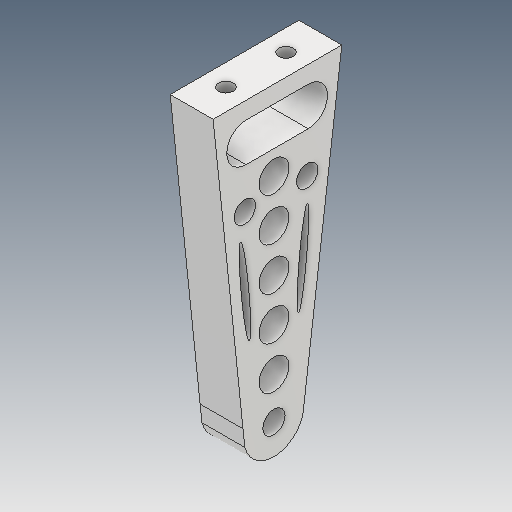
# Autodesk Inventor part: Radaufhängung
Saved by Autodesk Inventor 2018 (Build 220112000, 112)
## iProperties
Created: 2018-01-29
Part Number: Radaufhängung
Material: PC/ABS-Kunststoff
Document SubType Name: Modeling
Designer: Chris
Density: 0.357273 g/cm^3
Appearance: Schnee
Mass: 3.80196 g
Surface Area: 70.8958 cm^2
Volume: 10.6416 cm^3
Author: Chris
Autodesk Inventor part; units mm, degrees
note: some values were not read from the file. Chosen so that the rebuilt part matches the saved one: sketch regions of "Extrusion1".
ref_plane "YZ Plane" through (0, 0, 0) normal (1, 0, 0) x (0, 1, 0)
ref_plane "XZ Plane" through (0, 0, 0) normal (0, 1, 0) x (-1, 0, 0)
ref_plane "XY Plane" through (0, 0, 0) normal (0, 0, 1) x (1, 0, 0)
sketch "Skizze1" plane through (0, 0, 0) normal (1, 0, 0) x (0, 1, 0)
  line L0 (0, 0) -> (30, 0)
  line L1 (14.175552, 0) -> (14.175552, -68.187879) construction
  circle A0 centre (14.175552, -68.187879) radius 2.6
  circle A1 centre (14.175552, -68.187879) radius 7
  line L2 (0, 0) -> (7.179577, -67.95054)
  circle A2 centre (14.175552, -18.569993) radius 3.5
  arc A3 (7.675552, -4) -> (7.675552, -13) centre (7.675552, -8.5) ccw
  circle A4 centre (14.175552, -28.569993) radius 3.5
  circle A5 centre (14.175552, -38.569993) radius 3.5
  circle A6 centre (14.175552, -48.569993) radius 3.5
  circle A7 centre (14.175552, -58.569993) radius 3.5
  circle A8 centre (21.920836, -22.373144) radius 2.5
  circle A9 centre (7.389695, -22.35367) radius 2.5
  line L3 (7.675552, -4) -> (14.175552, -4)
  line L4 (7.675552, -13) -> (14.175552, -13)
  ellipse E0 centre (20.928749, -38.468301) end of major axis (19.90015, -48.968019) minor radius 0.865905
  ellipse E1 centre (7.422355, -38.468301) end of major axis (8.450954, -48.968019) minor radius 0.865905
  line L5 (21.175549, -68.194766) -> (30, 0)
  arc A10 (22.175552, -13) -> (22.175552, -4) centre (22.175552, -8.5) ccw
  line L6 (14.175552, -4) -> (22.175552, -4)
  line L7 (14.175552, -13) -> (22.175552, -13)
  point P0 (11.380257, -37.526628)
  point P1 (20.96203, -66.472155)
  dimension "d0" = 30
  dimension "d32" = 70
  dimension "d34" = 5.2
  dimension "d35" = 14
  dimension "d36" = 7
  dimension "d42" = 9
  dimension "d43" = 8.5
  dimension "d44" = 6.5
  dimension "d47" = 10
  dimension "d54" = 5
  dimension "d59" = 5
  dimension "d60" = 5
  dimension "d67" = 9
  dimension "d68" = 8
  constraints: 16 end point, 11 centre point, 7 point on circle, 4 point on line, 3 horizontal, 2 coincident, 2 parallel, 2 tangent, 2 vertical, 1 perpendicular, 1 symmetric about line, 12 other
  measures "d0" distance of L0.start L0.end
  measures "d32" distance of L0.end L1.end
  measures "d34" diameter of A0
  measures "d35" diameter of A1
  measures "d36" diameter of A2
  measures "d42" diameter of A3
  measures "d43" distance from line of L0 A3.centre
  measures "d44" distance from line of L1 A3.centre
  measures "d47" distance of A2.centre A4.centre
  measures "d54" diameter of A8
  measures "d59" diameter of A9
  measures "d60" distance from line of L2 A9.centre
  measures "d67" diameter of A10
  measures "d68" distance from line of L1 A10.centre
sketch "Skizze1 outline for Extrusion1" plane through (0, 0, 0) normal (1, 0, 0) x (0, 1, 0)
  circle A0 centre (14.175552, -58.569993) radius 3.5
  arc A1 (7.179577, -67.95054) -> (21.175549, -68.194766) centre (14.175552, -68.187879) ccw
  line L0 (21.175549, -68.194766) -> (30, 0)
  line L1 (30, 0) -> (0, 0)
  line L2 (0, 0) -> (7.179577, -67.95054)
  circle A2 centre (14.175552, -68.187879) radius 2.6
  arc A3 (22.175552, -13) -> (22.175552, -4) centre (22.175552, -8.5) ccw
  line L3 (22.175552, -13) -> (7.675552, -13)
  arc A4 (7.675552, -4) -> (7.675552, -13) centre (7.675552, -8.5) ccw
  line L4 (7.675552, -4) -> (22.175552, -4)
  circle A5 centre (14.175552, -48.569993) radius 3.5
  spline S0 degree 2 poles (8.450954, -48.968019) (9.9436, -48.821792) (7.654379, -33.14533) (5.365158, -17.468867) (6.161733, -33.291556) (6.958308, -49.114245) (8.450954, -48.968019) knots 0 0 0 0.33333333 0.33333333 0.66666667 0.66666667 1 1 1 weights 1 0.5 1 0.5 1 0.5 1
  circle A6 centre (14.175552, -38.569993) radius 3.5
  circle A7 centre (14.175552, -28.569993) radius 3.5
  spline S1 degree 2 poles (19.90015, -48.968019) (21.392796, -49.114245) (22.189371, -33.291556) (22.985946, -17.468867) (20.696725, -33.14533) (18.407504, -48.821792) (19.90015, -48.968019) knots 0 0 0 0.33333333 0.33333333 0.66666667 0.66666667 1 1 1 weights 1 0.5 1 0.5 1 0.5 1
  circle A8 centre (7.389695, -22.35367) radius 2.5
  circle A9 centre (14.175552, -18.569993) radius 3.5
  circle A10 centre (21.920836, -22.373144) radius 2.5
extrude "Extrusion1" add sketch "Skizze1 outline for Extrusion1" along normal blind 10
sketch "Skizze3" plane through (0, 0, 0) normal (0, 0, 1) x (1, 0, 0)
  circle A0 centre (5, 8) radius 1.7
  line L0 (0, 0) -> (10, 0) projected
  circle A1 centre (5, 22) radius 1.7
  line L1 (0, 30) -> (10, 30) projected
  line L2 (10, 30) -> (10, 0) projected
  dimension "d24" = 3.4
  dimension "d25" = 8
  dimension "d26" = 3.4
  dimension "d27" = 8
  dimension "d28" = 5
  constraints: 2 centre point
  measures "d24" diameter of A0
  measures "d25" distance from line of L0 A0.centre
  measures "d26" diameter of A1
  measures "d27" distance from line of L1 A1.centre
  measures "d28" distance from line of L2 A0.centre
sketch "Skizze3 outline for Extrusion2" plane through (0, 0, 0) normal (0, 0, 1) x (1, 0, 0)
  circle A0 centre (5, 8) radius 1.7
  circle A1 centre (5, 22) radius 1.7
extrude "Extrusion2" cut sketch "Skizze3 outline for Extrusion2" against normal blind 11
chamfer "Fase1" distance 2 angle 45 1 edges at (5, 7.1796, -67.9505)
chamfer "Fase3" distance 2 angle 45 1 edges at (5, 21.1755, -68.1948)
